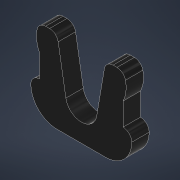
# Autodesk Inventor part: fastener_lock
Saved by Autodesk Inventor 2021 (Build 250183000, 183)
## iProperties
Created: 2021-01-30
Part Number: fastener_lock
Material: ABS Plastic
Document SubType Name: Modeling
Designer: User
Density: 1.06 g/cm^3
Appearance: Smooth - Black
Author: User
Autodesk Inventor part; units mm, degrees
ref_plane "YZ Plane" through (0, 0, 0) normal (1, 0, 0) x (0, 1, 0)
ref_plane "XZ Plane" through (0, 0, 0) normal (0, 1, 0) x (-1, 0, 0)
ref_plane "XY Plane" through (0, 0, 0) normal (0, 0, 1) x (1, 0, 0)
sketch "lock_sketch" plane through (0, 0, 0) normal (0, 0, 1) x (1, 0, 0)
  line L0 (0, 0) -> (10, 0) projected
  line L1 (10, 0) -> (10, 2.6) projected
  line L2 (0, 2.6) -> (10, 2.6) projected
  line L3 (0, 0) -> (0, 2.6) projected
  line L4 (0.2, -4) -> (9.8, -4) construction
  line L5 (9.8, -4) -> (9.8, 5.6) construction
  line L6 (9.8, 5.6) -> (0.2, 5.6)
  line L7 (0.2, 5.6) -> (0.2, -4) construction
  arc A0 (0.2, 5.6) -> (0.2, 2.6) centre (3.2, 4.1) ccw
  arc A1 (9.8, 2.6) -> (9.8, 5.6) centre (6.8, 4.1) ccw
  line L8 (5, -4) -> (5, 0) construction
  line L9 (9.8, 2.6) -> (9.8, 0)
  line L10 (0.2, 2.6) -> (0.2, 0)
  line L11 (0.2, 0) -> (0.2, 0)
  line L12 (-0.8, -1) -> (-0.8, -1)
  line L13 (2.2, -4) -> (7.8, -4)
  line L14 (10.8, -1) -> (10.8, -1)
  line L15 (9.8, 0) -> (9.8, 0)
  arc A2 (-0.8, -1) -> (2.2, -4) centre (2.2, -1) ccw
  arc A3 (7.8, -4) -> (10.8, -1) centre (7.8, -1) ccw
  arc A4 (0.2, 0) -> (-0.8, -1) centre (0.2, -1) ccw
  arc A5 (10.8, -1) -> (9.8, 0) centre (9.8, -1) ccw
  line L16 (2.2, 5.6) -> (3.5, -2)
  line L17 (3.5, -2) -> (6.5, -2)
  line L18 (6.5, -2) -> (7.8, 5.6)
  point P0 (-0.8, 0)
  point P1 (10.8, 0)
  point P2 (0.2, 0)
  point P3 (9.8, 0)
  point P4 (5, -4)
  dimension "d4" = 0
  dimension "d0" = 10
  dimension "d1" = 9.6
  dimension "d2" = 0.2
  dimension "d6" = 3
  dimension "d7" = 3
  dimension "d9" = 2
  dimension "d10" = 2
  dimension "d14" = 4
  dimension "d17" = 3
  dimension "d18" = 1
  dimension "d19" = 1
  dimension "d22" = 3
  dimension "d23" = 1
  dimension "d24" = 3
  dimension "d25" = 2
  constraints: 30 end point, 15 point on line, 12 point on circle, 8 tangent, 6 centre point, 5 horizontal, 4 perpendicular, 3 vertical, 2 equal radius, 2 horizontal alignment, 2 midpoint, 2 parallel, 1 collinear, 1 symmetric about line, 1 vertical alignment, 8 other
  measures "d0" distance of L2.start L1.end
  measures "d1" distance of L5.end L6.end
  measures "d2" distance between parallel lines of L3 L7
  measures "d6" distance between parallel lines of L2 L6
  measures "d7" distance from line of L5 A1.centre
  measures "d9" distance of L6.end L16.start
  measures "d10" distance of L5.end L18.end
  measures "d14" distance of L8.end L8.start
  measures "d17" distance from line of L7 A0.centre
  measures "d18" distance of L10.end point (-0.8, 0)
  measures "d19" distance of point (10.8, 0) L9.end
  measures "d22" radius of A2
  measures "d23" radius of A4
  measures "d24" distance of L16.end L17.end
  measures "d25" distance from line of L8.end L17
extrude "lock" add sketch "lock_sketch" along normal blind 2 contours L10 L2 L16 L0 | L0 L16 L17 L18 A5 A3 L13 A2 A4 | A0 L6 L16 L2 | L18 L2 L9 L0 | L18 L6 A1 L2
fillet "teeth" radius 1 4 edges at (2.2, 5.6, 1) (7.8, 5.6, 1) (0.2, 5.6, 1) (9.8, 5.6, 1)
fillet "inside" radius 1.8 2 edges at (3.5, -2, 1) (6.5, -2, 1)
equation "\"d2\" = -0.5 * d1 + 0.5 * d0"
equation "\"d7\" = d17"
equation "\"d19\" = d18"
equation "\"d25\" = 0.5 * d14"
body "Solid1"
